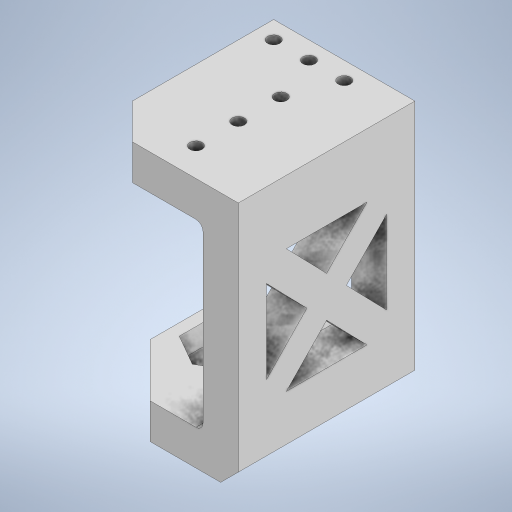
# Autodesk Inventor part: 전체 형상
Saved by Autodesk Inventor 2023 (Build 270158000, 158)
## iProperties
Created: 2022-11-11
Part Number: 전체 형상
Material: 일반
Document SubType Name: Modeling
Designer: hyunsu
Density: 1 g/cm^3
Appearance: 기본값
Author: hyunsu
Autodesk Inventor part; units mm, degrees
ref_plane "YZ Plane" through (0, 0, 0) normal (1, 0, 0) x (0, 1, 0)
ref_plane "XZ Plane" through (0, 0, 0) normal (0, 1, 0) x (-1, 0, 0)
sketch "스케치1" plane through (0, 0, 0) normal (0, 0, 1) x (1, 0, 0)
  line L0 (-5, -35.5) -> (5, -35.5)
  line L1 (5, -35.5) -> (5, 35.5)
  line L2 (5, 35.5) -> (-5, 35.5)
  line L3 (-5, 35.5) -> (-5, -35.5)
  line L4 (-5, -35.5) -> (5, 35.5) construction
  line L5 (5, -35.5) -> (-5, 35.5) construction
  line L6 (-5, 35.5) -> (-35, 35.5)
  line L7 (-35, 35.5) -> (-35, 25.5)
  line L8 (-35, 25.5) -> (-5, 25.5)
  line L9 (-5, 25.5) -> (-5, 35.5)
  line L10 (0, 0) -> (-11.0402, 0)
  line L11 (-5, -35.5) -> (-35, -35.5)
  line L12 (-35, -35.5) -> (-35, -25.5)
  line L13 (-35, -25.5) -> (-5, -25.5)
  point P0 (-5, 25.5)
  point P1 (-5, -25.5)
  dimension "d0" = 71
  dimension "d1" = 10
  dimension "d2" = 10
  dimension "d3" = 30
  constraints: 28 end point, 4 parallel, 3 horizontal, 3 symmetric about line, 2 midpoint, 2 perpendicular
  measures "d0" distance of L0.end L1.end
  measures "d1" distance of L1.end L2.end
  measures "d2" distance of L6.end L7.end
  measures "d3" distance of L2.end L6.end
extrude "돌출1" add sketch "스케치1" along normal mid plane 50
ref_plane "작업 평면1" through (-15, 25.5, -25) normal (-1, 0, 0) x (0, 0, 1)
sketch "스케치5" plane through (-5, -25.5, 25) normal (-1, 0, 0) x (0, 0, 1)
  line L0 (-50, 0) -> (0, 0) projected
  line L1 (0, 51) -> (0, 0) projected
  line L2 (-50, 51) -> (0, 51) projected
  line L3 (-50, 0) -> (-50, 51) projected
  line L4 (-8, 43) -> (-8, 8)
  line L5 (-8, 8) -> (-42, 8)
  line L6 (-42, 8) -> (-42, 43)
  line L7 (-42, 43) -> (-8, 43)
  line L8 (-42, 43) -> (-8, 8) construction
  line L9 (-36.4234, 43) -> (-8, 13.7406)
  line L10 (-42, 37.2594) -> (-13.5766, 8)
  line L11 (-25, 25.5) -> (-25, 37.0316)
  line L12 (-8, 43) -> (-42, 8) construction
  line L13 (-13.5766, 43) -> (-42, 13.7406)
  line L14 (-8, 37.2594) -> (-36.4234, 8)
  point P0 (-42, 13.7406)
  point P1 (-30.5766, 25.5)
  point P2 (-8, 37.2594)
  point P3 (-19.4234, 25.5)
  point P4 (-25, 19.7594)
  point P5 (-36.4234, 8)
  point P6 (-25, 31.2406)
  dimension "d24" = 8
  dimension "d25" = 4
  dimension "d26" = 4
  constraints: 22 end point, 4 point on line, 4 symmetric about line, 2 parallel, 1 vertical, 3 other
  measures "d24" distance between parallel lines of L2 L7
  measures "d25" distance between parallel lines of L8 L9
  measures "d26" distance between parallel lines of L8 L10
extrude "돌출5" cut sketch "스케치5" against normal blind 10 contours L4 L9 L14 | L13 L9 L7 | L10 L5 L14 | L13 L6 L10
fillet "모깎기1" radius 2 2 edges at (-5, 25.5, 0) (-5, -25.5, 0)
sketch "스케치6" plane through (-35, -35.5, 25) normal (0, -1, 0) x (1, 0, 0)
  circle A0 centre (12, -25) radius 5
  line L0 (0, -50) -> (0, 0) projected
  point P0 (35, -25)
  point P1 (0, -25)
  dimension "d30" = 10
  dimension "d31" = 12
  constraints: 1 centre point, 1 horizontal alignment, 1 midpoint
  measures "d30" diameter of A0
  measures "d31" distance from line of L0 A0.centre
extrude "돌출6" cut sketch "스케치6" against normal up to surface (10 mm away)
chamfer "모따기1" distance 15 angle 45 2 edges at (-35, -30.5, 25) (-35, -30.5, -25)
sketch "스케치7" plane through (-7, -25.5, 25) normal (0, 1, 0) x (1, 0, 0)
  circle A0 centre (-16, 25) radius 5 projected
  line L0 (-16, 35.0459) -> (-7.3, 30.0229)
  line L1 (-7.3, 30.0229) -> (-7.3, 19.9771)
  line L2 (-7.3, 19.9771) -> (-16, 14.9541)
  line L3 (-16, 14.9541) -> (-24.7, 19.9771)
  line L4 (-24.7, 19.9771) -> (-24.7, 30.0229)
  line L5 (-24.7, 30.0229) -> (-16, 35.0459)
  point P0 (7, 25)
  dimension "d37" = 17.4
  constraints: 12 end point, 1 coincident, 13 other
  measures "d37" distance between parallel lines of L1 L4
extrude "돌출7" cut sketch "스케치7" against normal blind 6 contours A0 | L0 L1 L2 L3 L4 L5
sketch "스케치14" plane through (-35, 25.5, -25) normal (0, -1, 0) x (1, 0, 0)
  circle A0 centre (5, 5) radius 1.75
  circle A1 centre (5, 5) radius 3
  line L0 (0, 0) -> (40, 0) projected
  line L1 (0, 0) -> (0, 50) projected
  circle A2 centre (15, 5) radius 1.75
  circle A3 centre (15, 5) radius 3
  circle A4 centre (25, 5) radius 1.75
  circle A5 centre (25, 5) radius 3
  point P0 (35, 25)
  dimension "d74" = 3.5
  dimension "d75" = 6
  dimension "d76" = 5
  dimension "d77" = 5
  dimension "d80" = 10
  constraints: 6 centre point, 3 coincident, 1 horizontal, 8 other
  measures "d74" diameter of A0
  measures "d75" diameter of A1
  measures "d76" distance from line of L0 A0.centre
  measures "d77" distance from line of L1 A0.centre
  measures "d80" distance of A0.centre A2.centre
extrude "돌출12" cut sketch "스케치14" against normal blind 10 contours A0 | A2 | A4
extrude "돌출13" cut sketch "스케치14" against normal blind 2.5 contours A1 | A3 | A4 | A5
sketch "스케치15" plane through (-35, 35.5, 25) normal (0, 1, 0) x (1, 0, 0)
  circle A0 centre (20, 8) radius 1.75
  line L0 (40, 0) -> (0, 0) projected
  line L1 (40, 50) -> (40, 0) projected
  circle A1 centre (20, 20) radius 1.75
  circle A2 centre (20, 32) radius 1.75
  point P0 (35, 25)
  point P1 (20, 0)
  dimension "d89" = 3.5
  dimension "d90" = 8
  dimension "d93" = 12
  constraints: 3 centre point, 1 midpoint, 1 vertical, 1 vertical alignment, 4 other
  measures "d89" diameter of A0
  measures "d90" distance from line of L0 A0.centre
  measures "d93" distance of A0.centre A1.centre
extrude "돌출14" cut sketch "스케치15" against normal up to surface (10 mm away)
chamfer "모따기3" distance 10 angle 45 1 edges at (-35, 30.5, 25)
chamfer "모따기4" distance 5 angle 45 1 edges at (5, -35.5, 0)
sketch "스케치16" plane through (-35, 25.5, -25) normal (0, -1, 0) x (1, 0, 0)
  circle A0 centre (20, 18) radius 1.75 projected
  circle A1 centre (20, 18) radius 3
  circle A2 centre (20, 30) radius 1.75 projected
  circle A3 centre (20, 30) radius 3
  circle A4 centre (20, 42) radius 1.75 projected
  circle A5 centre (20, 42) radius 3
  point P0 (35, 25)
  dimension "d106" = 6
  dimension "d107" = 6
  dimension "d108" = 6
  constraints: 3 centre point, 3 coincident
  measures "d106" diameter of A1
  measures "d107" diameter of A3
  measures "d108" diameter of A5
extrude "돌출15" cut sketch "스케치16" against normal blind 2.5 contours A0 | A1 | A2 | A3 | A4 | A5
